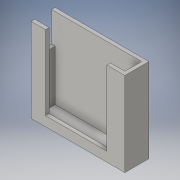
# Autodesk Inventor part: Phone Mount 2
Saved by Autodesk Inventor 2016 (Build 200138000, 138)
## iProperties
Created: 2016-01-15
Part Number: Phone Mount 2
Material: Generic
Document SubType Name: Modeling
Designer: TimB
Density: 1 g/cm^3
Appearance: Default
Author: TimB
Autodesk Inventor part; units mm, degrees
ref_plane "YZ Plane" through (0, 0, 0) normal (1, 0, 0) x (0, 1, 0)
ref_plane "XZ Plane" through (0, 0, 0) normal (0, 1, 0) x (-1, 0, 0)
ref_plane "XY Plane" through (0, 0, 0) normal (0, 0, 1) x (1, 0, 0)
sketch "Sketch1" plane through (0, 0, 0) normal (0, 1, 0) x (-1, 0, 0)
  line L0 (-7, -36) -> (7, -36)
  line L1 (7, -36) -> (7, 36)
  line L2 (7, 36) -> (-7, 36)
  line L3 (-7, 36) -> (-7, -36)
  line L4 (-7, -36) -> (7, 36) construction
  line L5 (7, -36) -> (-7, 36) construction
  line L6 (-10, -39) -> (10, -39)
  line L7 (10, -39) -> (10, 39)
  line L8 (10, 39) -> (-10, 39)
  line L9 (-10, 39) -> (-10, -39)
  line L10 (-10, -39) -> (10, 39) construction
  line L11 (10, -39) -> (-10, 39) construction
  point P0 (0, 0)
  dimension "d0" = 14
  dimension "d1" = 72
  dimension "d2" = 20
  dimension "d3" = 78
  constraints: 24 end point, 4 midpoint, 4 parallel, 2 horizontal, 2 perpendicular
  measures "d0" distance of L2.end L1.end
  measures "d1" distance of L1.end L0.end
  measures "d2" distance of L8.end L7.end
  measures "d3" distance of L7.end L6.end
extrude "Extrusion1" add sketch "Sketch1" along normal blind 42
sketch "Sketch2" plane through (10, 0, 39) normal (1, 0, 0) x (0, 0, -1)
  line L0 (78, 42) -> (0, 42) projected
  line L1 (12, 5) -> (63, 5)
  line L2 (12, 5) -> (12, 42)
  line L3 (63, 5) -> (63, 42)
  point P0 (39, 0)
  point P1 (39, 42)
  dimension "d6" = 78
  dimension "d7" = 51
  constraints: 6 end point, 2 point on line, 1 midpoint, 1 perpendicular, 1 vertical
  measures "d6" distance of L0.start L0.end
  measures "d7" distance of L1.end L1.start
extrude "Extrusion2" cut sketch "Sketch2" against normal blind 10
sketch "Sketch3" plane through (0, 42, 0) normal (0, 1, 0) x (1, 0, 0)
  line L0 (-10, 39) -> (-10, -39) projected
  line L1 (10, 39) -> (-10, 39) projected
  line L2 (10, 24) -> (10, 39) projected
  line L3 (-7, 36) -> (7, 36) projected
  line L4 (7, 36) -> (7, 24) projected
  line L5 (7, 24) -> (10, 24) projected
  line L6 (10, -39) -> (10, -27) projected
  line L7 (10, -27) -> (7, -27) projected
  line L8 (-7, 36) -> (-7, -36) projected
  line L9 (-7, -39) -> (-7, 36)
  line L10 (-10, -39) -> (-7, -39)
  line L11 (7, -39) -> (7, -27)
  line L12 (10, -39) -> (7, -39)
  point P0 (0, 0)
  constraints: 8 end point, 1 collinear
extrude "Extrusion3" add sketch "Sketch3" along normal blind 25
sketch "Sketch4" plane through (0, 0, 0) normal (0, -1, 0) x (1, 0, 0)
  line L0 (10, 39) -> (10, -39) projected
  line L1 (-10, 39) -> (10, 39) projected
  line L2 (-10, -39) -> (-10, 39) projected
  line L3 (10, -39) -> (-10, -39) projected
  point P0 (0, 0)
extrude "Extrusion4" add sketch "Sketch4" along normal blind 3
body "Solid1"
